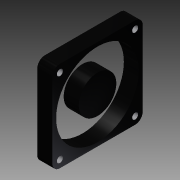
# Autodesk Inventor part: fan_60
Saved by Autodesk Inventor 2013 (Build 170138000, 138)
## iProperties
Created: 2013-06-08
Part Number: fan_60
Material: Generic
Document SubType Name: Modeling
Designer: dzban
Density: 1 g/cm^3
Author: dzban
Autodesk Inventor part; units mm, degrees
ref_plane "YZ Plane" through (0, 0, 0) normal (1, 0, 0) x (0, 1, 0)
ref_plane "XZ Plane" through (0, 0, 0) normal (0, 1, 0) x (-1, 0, 0)
ref_plane "XY Plane" through (0, 0, 0) normal (0, 0, 1) x (1, 0, 0)
sketch "Sketch1" plane through (0, 0, 0) normal (1, 0, 0) x (0, 1, 0)
  line L0 (5, 0) -> (55, 0)
  line L1 (60, 5) -> (60, 55)
  line L2 (55, 60) -> (5, 60)
  line L3 (0, 55) -> (0, 5)
  arc A0 (5, 60) -> (0, 55) centre (5, 55) ccw
  arc A1 (0, 5) -> (5, 0) centre (5, 5) ccw
  arc A2 (60, 55) -> (55, 60) centre (55, 55) ccw
  arc A3 (55, 0) -> (60, 5) centre (55, 5) ccw
  circle A4 centre (5, 55) radius 2
  circle A5 centre (5, 5) radius 2
  circle A6 centre (55, 5) radius 2
  circle A7 centre (55, 55) radius 2
  circle A8 centre (30, 30) radius 27.5
  circle A9 centre (30, 30) radius 12.4881
  point P0 (0, 0)
  point P1 (60, 60)
  point P2 (60, 0)
  point P3 (0, 60)
  dimension "d0" = 60
  dimension "d2" = 60
  dimension "d3" = 5
  dimension "d4" = 5
  dimension "d5" = 4
  dimension "d6" = 4
  dimension "d7" = 4
  dimension "d8" = 4
  dimension "d9" = 30
  dimension "d10" = 30
  dimension "d11" = 55
  constraints: 10 centre point, 8 end point, 8 point on circle, 8 point on line, 8 tangent, 5 coincident, 2 equal radius, 2 parallel, 1 horizontal, 1 perpendicular
  measures "d0" distance of point (60, 60) point (0, 60)
  measures "d2" distance of point (60, 0) point (60, 60)
  measures "d3" radius of A0
  measures "d4" radius of A1
  measures "d5" diameter of A4
  measures "d6" diameter of A5
  measures "d7" diameter of A6
  measures "d8" diameter of A7
  measures "d9" distance from line of L2 A8.centre
  measures "d10" distance from line of L3 A8.centre
  measures "d11" diameter of A8
extrude "Extrusion1" add sketch "Sketch1" along normal blind 10
body "Solid1"
